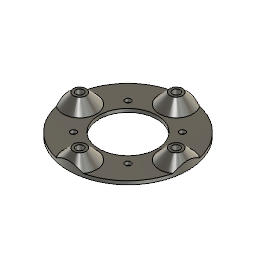
RingBottom (Autodesk Fusion 360 design; units mm, degrees)
Autodesk Fusion 360 part; units mm, degrees
sketch "Sketch1" plane through (0, 0, 0) normal (0, 0, 1) x (-1, 0, 0)
  circle A0 centre (0, 0) radius 34
  line L0 (0, -34) -> (0, -27.45) construction
  circle A1 centre (0, -27.45) radius 2.15
  circle A2 centre (0, -27.45) radius 3.6
  circle A3 centre (27.45, 0) radius 3.6
  circle A4 centre (27.45, 0) radius 2.15
  circle A5 centre (0, 27.45) radius 3.6
  circle A6 centre (0, 27.45) radius 2.15
  circle A7 centre (-27.45, 0) radius 3.6
  circle A8 centre (-27.45, 0) radius 2.15
  line L1 (0, 0) -> (0, -27.45) construction
  circle A9 centre (0, 0) radius 16.5
  line L2 (0, 0) -> (-15.4998, -15.4998) construction
  line L3 (0, 0) -> (21.92, 0) construction
  circle A10 centre (-15.4998, -15.4998) radius 1.65
  circle A11 centre (15.4998, -15.4998) radius 1.65
  circle A12 centre (15.4998, 15.4998) radius 1.65
  circle A13 centre (-15.4998, 15.4998) radius 1.65
  dimension "d12" = 68
  dimension "d22" = 4.3
  dimension "d24" = 7.2
  dimension "d26" = 360
  dimension "d35" = 27.45
  dimension "d53" = 33
  dimension "d54" = 135
  dimension "d55" = 21.92
  dimension "d56" = 3.3
  dimension "d58" = 360
  constraint coincident A0.centre L1.start
  constraint coincident A0 L0.start
  constraint vertical L0
  constraint coincident L0.end A1.centre
  constraint concentric A1 A2
  constraint parallel L0 L1
  constraint horizontal L3
  constraint coincident L2.end A10.centre
  measures "d12" diameter of A0
  measures "d22" diameter of A1
  measures "d24" diameter of A2
  measures "d35" distance of A0.centre L0.end
  measures "d53" diameter of A9
  measures "d54" angle of L2 L3
  measures "d55" distance of A0.centre L2.end
  measures "d56" diameter of A10
extrude "Extrude1" add sketch "Sketch1" along normal blind 2 contours A0 | A2 | A3 | A5 | A7
extrude "Extrude2" add sketch "Sketch1" along normal blind 6 from surface at 2 contours A2 | A3 | A5 | A7
chamfer "Chamfer1" distance 6 angle 45 4 edges at (3.3564, 26.1482, 2) (-24.0936, -1.3018, 2) (3.3564, -28.7518, 2) (30.8064, -1.3018, 2)
equation "gear_ratio = 6"
equation "gear_Ns = if(is_Nema_17 == 1; 12; 15)"
equation "gear_Nr = ( gear_ratio - 1 ) * gear_Ns"
equation "gear_OD = ( gear_Nr * diameter_scale * module ) + wall_thickness"
equation "thickness = 2 mm"
equation "m3_pilot = 3.3 mm"
equation "d12 = gear_OD"
equation "d17 = thickness"
equation "m3_inserts = 4.3 mm"
equation "m3_inserts_wall_thickness = 2.9 mm"
equation "d22 = m3_inserts"
equation "d24 = m3_inserts + m3_inserts_wall_thickness"
equation "m3_inserts_wall_height = 6 mm"
equation "d29 = m3_inserts_wall_height"
equation "d31 = m3_inserts_wall_chamfer"
equation "m3_inserts_wall_chamfer = 6 mm"
equation "m3_inserts_distance_from_center = 27.45 mm"
equation "d35 = m3_inserts_distance_from_center"
equation "motor_base_diameter = ( if(is_Nema_17 == 1; 33; 40) ) * 1 mm"
equation "d53 = motor_base_diameter"
equation "d55 = mount_holes_distance_from_center"
equation "d56 = mount_holes_diameter"
equation "mount_holes_distance_from_center = ( if(is_Nema_17 == 1; 21.92; 33.333) ) * 1 mm"
equation "mount_holes_diameter = if(is_Nema_17 == 1; m3_pilot; m45_pilot)"
equation "is_Nema_17 = 1"
equation "m45_pilot = 4.8 mm"
equation "helix_angle = 0 deg"
equation "diameter_scale = ( 1 / cos(helix_angle) ) * 1 mm"
equation "wall_thickness = 8 mm"
equation "module = 1"
